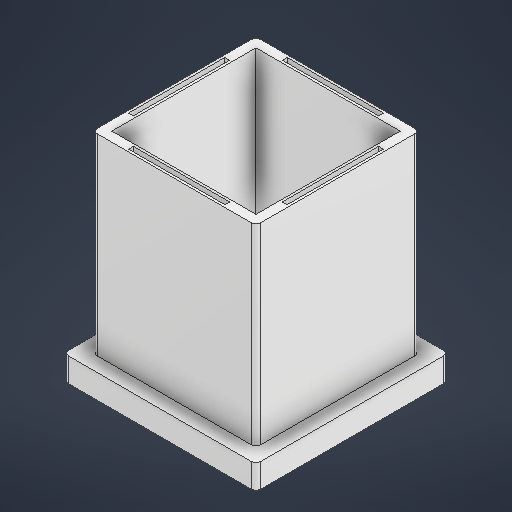
# Autodesk Inventor part: block_main
Saved by Autodesk Inventor 2025.2 (Build 292293000, 293)
## iProperties
Created: 2025-08-04
Part Number: block_main
Material: PC/ABS Plastic
Document SubType Name: Modeling
Designer: sam
Density: 1.1 g/cm^3
Appearance: Smooth - White
Author: sam
Autodesk Inventor part; units mm, degrees
ref_plane "YZ Plane" through (0, 0, 0) normal (1, 0, 0) x (0, 1, 0)
ref_plane "XZ Plane" through (0, 0, 0) normal (0, 1, 0) x (-1, 0, 0)
ref_plane "XY Plane" through (0, 0, 0) normal (0, 0, 1) x (1, 0, 0)
sketch "Sketch1" plane through (0, 0, 0) normal (0, 1, 0) x (-1, 0, 0)
  line L0 (-20, -20) -> (20, -20)
  line L1 (20, -20) -> (20, 20)
  line L2 (20, 20) -> (-20, 20)
  line L3 (-20, 20) -> (-20, -20)
  line L4 (-20, -20) -> (20, 20) construction
  line L5 (20, -20) -> (-20, 20) construction
  point P0 (0, 0)
  dimension "d2" = 40
  dimension "d3" = 40
  constraints: 12 end point, 2 midpoint, 2 parallel, 1 horizontal, 1 perpendicular
  measures "d2" distance of L2.end L1.end
  measures "d3" distance of L1.end L0.end
extrude "Extrusion1" add sketch "Sketch1" along normal blind 5
sketch "Sketch2" plane through (0, 5, 0) normal (0, 1, 0) x (1, 0, 0)
  line L0 (-20, 20) -> (-20, -20) projected
  line L1 (-20, -20) -> (20, -20) projected
  line L2 (20, -20) -> (20, 20) projected
  line L3 (20, 20) -> (-20, 20) projected
  line L4 (17, 17) -> (-17, 17)
  line L5 (-17, 17) -> (-17, -17)
  line L6 (-17, -17) -> (17, -17)
  line L7 (17, -17) -> (17, 17)
  line L8 (17, 17) -> (-17, -17) construction
  line L9 (-17, 17) -> (17, -17) construction
  line L10 (15, 15) -> (-15, 15)
  line L11 (-15, 15) -> (-15, -15)
  line L12 (-15, -15) -> (15, -15)
  line L13 (15, -15) -> (15, 15)
  line L14 (15, 15) -> (-15, -15) construction
  line L15 (-15, 15) -> (15, -15) construction
  point P0 (0, 0)
  dimension "d6" = 3
  dimension "d7" = 2
  dimension "d52" = 3
  dimension "d53" = 2
  constraints: 24 end point, 4 midpoint, 4 parallel, 2 horizontal, 1 perpendicular
  measures "d6" distance between parallel lines of L0 L5
  measures "d7" distance between parallel lines of L6 L12
  measures "d52" distance between parallel lines of L1 L6
  measures "d53" distance between parallel lines of L5 L11
extrude "Extrusion2" add sketch "Sketch2" along normal blind 40 contours L7 L6 L5 L4
fillet "Fillet1" radius 1 1 edges at (20, 2.5, 20)
fillet "Fillet2" radius 1 1 edges at (20, 2.5, -20)
fillet "Fillet3" radius 1 1 edges at (-20, 2.5, 20)
fillet "Fillet4" radius 1 1 edges at (-20, 2.5, -20)
fillet "Fillet5" radius 1 1 edges at (-17, 25, 17)
fillet "Fillet6" radius 1 1 edges at (17, 25, 17)
fillet "Fillet7" radius 1 1 edges at (17, 25, -17)
fillet "Fillet8" radius 1 1 edges at (-17, 25, -17)
sketch "Sketch3" plane through (0, 45, 0) normal (0, 1, 0) x (1, 0, 0)
  arc A0 (-16, 17) -> (-17, 16) centre (-16, 16) ccw projected
  line L0 (-17, 16) -> (-17, -16) projected
  arc A1 (-17, -16) -> (-16, -17) centre (-16, -16) ccw projected
  line L1 (-16, -17) -> (16, -17) projected
  arc A2 (16, -17) -> (17, -16) centre (16, -16) ccw projected
  line L2 (17, -16) -> (17, 16) projected
  arc A3 (17, 16) -> (16, 17) centre (16, 16) ccw projected
  line L3 (16, 17) -> (-16, 17) projected
  line L4 (15, 15) -> (15, -15) projected
  line L5 (15, -15) -> (-15, -15) projected
  line L6 (-15, -15) -> (-15, 15) projected
  line L7 (-15, 15) -> (15, 15) projected
  line L8 (-16.5, -10) -> (-15.5, -10)
  line L9 (-15.5, -10) -> (-15.5, 10)
  line L10 (-15.5, 10) -> (-16.5, 10)
  line L11 (-16.5, 10) -> (-16.5, -10)
  line L12 (-16.5, 10) -> (-15.5, 10)
  line L13 (-15.5, 10) -> (-15.5, -10)
  line L14 (-15.5, -10) -> (-16.5, -10)
  line L15 (-16.5, -10) -> (-16.5, 10)
  line L16 (-10, 16.5) -> (10, 16.5)
  line L17 (10, 16.5) -> (10, 15.5)
  line L18 (10, 15.5) -> (-10, 15.5)
  line L19 (-10, 15.5) -> (-10, 16.5)
  line L20 (10, 16.5) -> (-10, 16.5)
  line L21 (-10, 16.5) -> (-10, 15.5)
  line L22 (-10, 15.5) -> (10, 15.5)
  line L23 (10, 15.5) -> (10, 16.5)
  line L24 (15.5, 10) -> (16.5, 10)
  line L25 (16.5, 10) -> (16.5, -10)
  line L26 (16.5, -10) -> (15.5, -10)
  line L27 (15.5, -10) -> (15.5, 10)
  line L28 (15.5, -10) -> (16.5, -10)
  line L29 (16.5, -10) -> (16.5, 10)
  line L30 (16.5, 10) -> (15.5, 10)
  line L31 (15.5, 10) -> (15.5, -10)
  line L32 (10, -15.5) -> (-10, -15.5)
  line L33 (-10, -15.5) -> (-10, -16.5)
  line L34 (-10, -16.5) -> (10, -16.5)
  line L35 (10, -16.5) -> (10, -15.5)
  line L36 (-10, -15.5) -> (10, -15.5)
  line L37 (10, -15.5) -> (10, -16.5)
  line L38 (10, -16.5) -> (-10, -16.5)
  line L39 (-10, -16.5) -> (-10, -15.5)
  point P0 (0, 0)
  point P1 (-16, 10)
  point P2 (-16, -10)
  point P3 (16, 10)
  dimension "d18" = 1
  dimension "d19" = 20
  dimension "d20" = 0.5
  dimension "d21" = 7
  dimension "d22" = 7
  dimension "d23" = 0.5
  dimension "d24" = 1
  dimension "d25" = 20
  dimension "d26" = 20
  dimension "d27" = 1
  dimension "d28" = 0.5
  dimension "d29" = 7
  dimension "d30" = 20
  dimension "d31" = 1
  dimension "d32" = 0.5
  dimension "d33" = 7
  dimension "d34" = 1
  dimension "d35" = 20
  dimension "d36" = 0.5
  dimension "d37" = 7
  dimension "d38" = 1
  dimension "d39" = 20
  dimension "d40" = 7
  dimension "d41" = 0.5
  dimension "d42" = 20
  dimension "d43" = 1
  dimension "d44" = 0.5
  dimension "d45" = 7
  dimension "d46" = 20
  dimension "d47" = 1
  dimension "d48" = 0.5
  dimension "d49" = 7
  constraints: 64 end point, 14 parallel, 7 horizontal, 7 perpendicular, 3 midpoint
  measures "d18" distance of L10.end L9.end
  measures "d19" distance of L9.end L8.end
  measures "d20" distance between parallel lines of L0 L11
  measures "d21" distance between parallel lines of L8 L1
  measures "d22" distance between parallel lines of L3 L12
  measures "d23" distance between parallel lines of L0 L15
  measures "d24" distance between parallel lines of L13 L15
  measures "d25" distance of point (-16, 10) point (-16, -10)
  measures "d26" distance of L17.end L18.end
  measures "d27" distance of L16.end L17.end
  measures "d28" distance between parallel lines of L3 L16
  measures "d29" distance between parallel lines of L0 L19
  measures "d30" distance of L22.end L21.end
  measures "d31" distance of L21.end L20.end
  measures "d32" distance between parallel lines of L3 L20
  measures "d33" distance between parallel lines of L2 L23
  measures "d34" distance of L25.end L26.end
  measures "d35" distance of L24.end L25.end
  measures "d36" distance between parallel lines of L2 L25
  measures "d37" distance from line of L3 point (16, 10)
  measures "d38" distance of L30.end L29.end
  measures "d39" distance of L29.end L28.end
  measures "d40" distance between parallel lines of L1 L28
  measures "d41" distance between parallel lines of L2 L29
  measures "d42" distance of L34.end L33.end
  measures "d43" distance of L33.end L32.end
  measures "d44" distance between parallel lines of L1 L34
  measures "d45" distance between parallel lines of L2 L35
  measures "d46" distance of L37.end L38.end
  measures "d47" distance of L36.end L37.end
  measures "d48" distance between parallel lines of L1 L38
  measures "d49" distance from line of L0 L36.start
extrude "Extrusion3" cut sketch "Sketch3" against normal blind 1 contours L11 L10 L9 L8 | L16 L17 L18 L19 | L24 L25 L26 L27 | L35 L34 L33 L32
body "Solid1"
